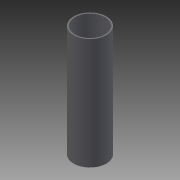
# Autodesk Inventor part: 022.08-FO1_BM_tube
Saved by Autodesk Inventor 2014 (Build 180170000, 170)
## iProperties
Created: 2014-01-19
Part Number: 022.08-FO1_BM_tube
Material: Steel
Catalog Web Link: www.cadenas.de
Description: FO1_basic_model_tube-Bimba FLAT-1
Vendor: BIMBA
Document SubType Name: Standard Catalog Part
Designer: Andrew Toennies
Manufacturer: BIMBA
Density: 1 g/cm^3
Appearance: Steel
Category: PARTsolutions
Company: BIMBA
PSOL_IDENT_0: {$CADENAS_DATA\23d-libs\bimba\bimba\bimba_imperial\bimba_full_line\flat_cylinders\fo1\fo1_basic_mode
PSOL_IDENT_1: l_tube.prj},198 {VTYP=3D},{NB=022.08-FO1_BM_tube},{LINA=022.08-FO1_BM_tube},{NN=FO1_basic_model_tube
PSOL_IDENT_2: },{DATE=08.09.2011 08:17:06},{GEOMDATE=08.09.2011 08:17:00},{VERSION=},{LINEID=10},{LINESUBID=-1},{W
PSOL_IDENT_3: BVAR=STROKE}  {NB=022.08-FO1_BM_tube},{LINA=022.08-FO1_BM_tube},{KT=DUMMY},{PN=022.08-FO1_BM_tube},{
PSOL_IDENT_4: BORE=0.56250000},{BOREPN=02},{STROKE=2.08},{STROKEMIN=0.202},{A=1.12000000},{BA=0.56000},{BB=0.69000
PSOL_IDENT_5: },{BC=1.96},{BD=2.14},{C=0.88000000},{DD=2.00000000},{D=0.11200000},{CPIL=0.12000000},{DC=0.18800000
PSOL_IDENT_6: },{DCP=0.12000000},{DCD=0.85500000},{ES=0.16400000},{EC=0.00000000},{ED=0.46000000},{F=0.25000000},{
PSOL_IDENT_7: H=0.22000000},{J=0.34000000},{K=0.14000000},{L=0.19000000},{LDP=0.20000000},{LP=0.16000000},{LPDP=0.
PSOL_IDENT_8: 28000000},{TD=0.65700000},{TDDP=0.10000},{TD1=0.59500},{TD2=0.61000},{TDIN=0.56200},{LSF=0.31250000}
PSOL_IDENT_9: ,{LSFDP=0.02000000},{BC1=0.81000},{BC2=1.38000},{BC3=1.96000},{BC4=2.52000},{BD1=1.06000},{BD2=1.620
PSOL_IDENT_10: 00},{BD3=2.14000},{BD4=2.70000}
CNS_NN: FO1_basic_model_tube
CNS_NT: Bimba FLAT-1
CNS_NB: 022.08-FO1_BM_tube
CNS_NBSYN: $PN.
CNS_LINA: 022.08-FO1_BM_tube
CNS_PN: 022.08-FO1_BM_tube
CNS_BORE: 9/16
CNS_BOREPN: 02
CNS_STROKE: 2.080
CNS_STROKEMIN: 0.202
CNS_A: 1.12000000
CNS_BA: 0.56000
CNS_BB: 0.69000
CNS_BC: 1.960
CNS_BD: 2.140
CNS_C: 0.88000000
CNS_DD: 2.00000000
CNS_D: 0.11200000
CNS_CPIL: 0.12000000
CNS_DC: 0.18800000
CNS_DCP: 0.12000000
CNS_DCD: 0.85500000
CNS_ES: 0.16400000
CNS_EC: 0.00000000
CNS_ED: 0.46000000
CNS_F: 0.25000000
CNS_H: 0.22000000
CNS_J: 0.34000000
CNS_K: 0.14000000
CNS_L: 0.19000000
CNS_LDP: 0.20000000
CNS_LP: 0.16000000
CNS_LPDP: 0.28000000
CNS_TD: 0.65700000
CNS_TDDP: 0.10000
CNS_TD1: 0.59500
CNS_TD2: 0.61000
CNS_TDIN: 0.56200
CNS_LSF: 0.31250000
CNS_LSFDP: 0.02000000
CNS_BC1: 0.81000
CNS_BC2: 1.38000
CNS_BC3: 1.96000
CNS_BC4: 2.52000
CNS_BD1: 1.06000
CNS_BD2: 1.62000
CNS_BD3: 2.14000
CNS_BD4: 2.70000
SUPPLIER: BIMBA
ARTICLENO: 022.08-FO1_BM_tube
BOMINFO: 022.08-FO1_BM_tube
CREATOR: CADENAS GmbH
Title: 022.08-FO1_BM_tube
Author: Cadenas PARTsolutions
Comments: Bimba FLAT-1
Autodesk Inventor part; units mm, degrees
ref_plane "YZ Plane" through (0, 0, 0) normal (1, 0, 0) x (0, 1, 0)
ref_plane "XZ Plane" through (0, 0, 0) normal (0, 1, 0) x (-1, 0, 0)
ref_plane "XY Plane" through (0, 0, 0) normal (0, 0, 1) x (1, 0, 0)
sketch "Sketch_4" plane through (0, 0, 0) normal (0, 0, 1) x (1, 0, 0)
  line L0 (0, 0) -> (0, 52.832)
  line L1 (7.1374, 0) -> (7.747, 0)
  line L2 (7.747, 0) -> (7.747, 52.832)
  line L3 (7.747, 52.832) -> (7.1374, 52.832)
  line L4 (7.1374, 52.832) -> (7.1374, 0)
  constraints: 10 end point
revolve "Revolution1" add sketch "Sketch_4" angle 360 about axis through (0, 0, 0) along (0, -1, 0)
ref_plane "tube_rear_XY" through (0, 52.832, 0) normal (0, 1, 0) x (1, 0, 0)
ref_plane "tube_rear_YZ" through (0, 52.832, 0) normal (1, 0, 0) x (0, 0, -1)
ref_plane "tube_rear_ZX" through (0, 52.832, 0) normal (0, 0, -1) x (0, 1, 0)
ref_plane "tube_rod_guide_XY" through (0, 0, 0) normal (0, 1, 0) x (1, 0, 0)
ref_plane "tube_rod_guide_YZ" through (0, 0, 0) normal (1, 0, 0) x (0, 0, -1)
ref_plane "tube_rod_guide_ZX" through (0, 0, 0) normal (0, 0, -1) x (0, 1, 0)
body "Solid1"
